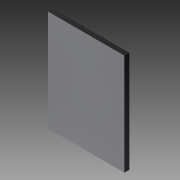
# Autodesk Inventor part: Field
Saved by Autodesk Inventor 2015 (Build 190159000, 159)
## iProperties
Created: 2016-02-20
Part Number: Field
Material: Generic
Document SubType Name: Modeling
Designer: 23902
Density: 1 g/cm^3
Appearance: Default
Author: 23902
Autodesk Inventor part; units mm, degrees
ref_plane "YZ Plane" through (0, 0, 0) normal (1, 0, 0) x (0, 1, 0)
ref_plane "XZ Plane" through (0, 0, 0) normal (0, 1, 0) x (-1, 0, 0)
ref_plane "XY Plane" through (0, 0, 0) normal (0, 0, 1) x (1, 0, 0)
sketch "Sketch1" plane through (0, 0, 0) normal (0, 1, 0) x (-1, 0, 0)
  line L0 (-910, 1215) -> (910, 1215)
  line L1 (910, 1215) -> (910, -1215)
  line L2 (910, -1215) -> (-910, -1215)
  line L3 (-910, -1215) -> (-910, 1215)
  line L4 (-910, 1215) -> (910, -1215) construction
  line L5 (910, 1215) -> (-910, -1215) construction
  point P0 (0, 0)
  dimension "d0" = 1820
  dimension "d1" = 2430
  constraints: 12 end point, 2 midpoint, 2 parallel, 1 horizontal, 1 perpendicular
  measures "d0" distance of L0.start L0.end
  measures "d1" distance of L0.end L1.end
extrude "Extrusion1" add sketch "Sketch1" along normal blind 20
sketch "Sketch2" plane through (0, 20, 0) normal (0, 1, 0) x (1, 0, 0)
  point P0 (0, 0)
sketch "Sketch3" plane through (0, 0, 0) normal (0, -1, 0) x (1, 0, 0)
  line L0 (910, 1215) -> (-910, 1215) projected
  line L1 (-910, 1215) -> (-910, -1215) projected
  line L2 (-910, -1215) -> (910, -1215) projected
  line L3 (910, -1215) -> (910, 1215) projected
  line L4 (910, 1215) -> (910, 1235)
  line L5 (910, 1235) -> (930, 1235)
  line L6 (-910, -1215) -> (-930, -1215)
  line L7 (-930, -1215) -> (-930, -1235)
  line L8 (-930, -1235) -> (930, -1235)
  line L9 (930, -1235) -> (930, 1235)
  line L10 (930, 1235) -> (-930, 1235)
  line L11 (-930, 1235) -> (-930, -1235)
  point P0 (0, 0)
  dimension "d4" = 20
  dimension "d5" = 20
  dimension "d6" = 20
  dimension "d7" = 20
  constraints: 16 end point, 3 perpendicular, 2 horizontal, 2 parallel, 1 vertical
  measures "d4" distance of L0.start L4.end
  measures "d5" distance of L4.end L5.end
  measures "d6" distance of L1.end L6.end
  measures "d7" distance of L6.end L7.end
extrude "Extrusion2" add sketch "Sketch3" against normal blind 120 contours L4 L5 L9 L8 L7 L6 L2 L3 | L0 L1 L6 L11 L10 L4
sketch "Sketch6" plane through (0, 20, 0) normal (0, 1, 0) x (1, 0, 0)
  line L0 (910, -1215) -> (-910, -1215) projected
  line L1 (225, -915) -> (245, -915)
  line L2 (245, -915) -> (245, -1215)
  line L3 (225, -915) -> (225, -989)
  line L4 (225, -989) -> (-225, -989)
  line L5 (-225, -1215) -> (-245, -1215)
  line L6 (-245, -1215) -> (-245, -915)
  line L7 (-245, -915) -> (-225, -915)
  line L8 (-225, -915) -> (-225, -989)
  line L9 (-225, -1009) -> (225, -1009)
  line L10 (225, -1009) -> (225, -1215)
  line L11 (-225, -1009) -> (-225, -1215)
  line L12 (245, -1215) -> (225, -1215)
  line L13 (225, 915) -> (245, 915)
  line L14 (245, 915) -> (245, 1215)
  line L15 (225, 915) -> (225, 989)
  line L16 (225, 989) -> (-225, 989)
  line L17 (-225, 1215) -> (-245, 1215)
  line L18 (-245, 1215) -> (-245, 915)
  line L19 (-245, 915) -> (-225, 915)
  line L20 (-225, 915) -> (-225, 989)
  line L21 (-225, 1009) -> (225, 1009)
  line L22 (225, 1009) -> (225, 1215)
  line L23 (-225, 1009) -> (-225, 1215)
  line L24 (245, 1215) -> (225, 1215)
  point P0 (0, 0)
  dimension "d22" = 20
  dimension "d23" = 74
  dimension "d24" = 450
  dimension "d25" = 20
  dimension "d26" = 20
  constraints: 48 end point, 5 perpendicular, 4 point on line, 3 vertical, 1 collinear, 1 parallel
  measures "d22" distance of L1.start L1.end
  measures "d23" distance of L1.start L3.end
  measures "d24" distance of L3.end L4.end
  measures "d25" distance of L5.start L5.end
  measures "d26" distance of L4.end L9.start
extrude "Extrusion3" add sketch "Sketch6" along normal blind 140 contours L0 L10 L9 L11 L6 L7 L8 L4 L3 L1 L2 | L15 L16 L20 L19 L18 L17 L23 L21 L22 L24 L14 L13
sketch "Sketch7" plane through (0, 160, 0) normal (0, 1, 0) x (1, 0, 0)
  line L0 (225, -915) -> (225, -989) projected
  line L1 (225, -989) -> (-225, -989) projected
  line L2 (-225, -989) -> (-225, -915) projected
  line L3 (-225, -915) -> (-245, -915) projected
  line L4 (-245, -915) -> (-245, -1215) projected
  line L5 (-245, -1215) -> (-225, -1215) projected
  line L6 (-225, -1215) -> (-225, -1009) projected
  line L7 (-225, -1009) -> (225, -1009) projected
  line L8 (225, -1009) -> (225, -1215) projected
  line L9 (225, -1215) -> (245, -1215) projected
  line L10 (245, -1215) -> (245, -915) projected
  line L11 (245, -915) -> (225, -915) projected
  line L12 (-225, 989) -> (225, 989) projected
  line L13 (225, 989) -> (225, 915) projected
  line L14 (225, 915) -> (245, 915) projected
  line L15 (245, 915) -> (245, 1215) projected
  line L16 (245, 1215) -> (225, 1215) projected
  line L17 (225, 1215) -> (225, 1009) projected
  line L18 (225, 1009) -> (-225, 1009) projected
  line L19 (-225, 1009) -> (-225, 1215) projected
  line L20 (-225, 1215) -> (-245, 1215) projected
  line L21 (-245, 1215) -> (-245, 915) projected
  line L22 (-245, 915) -> (-225, 915) projected
  line L23 (-225, 915) -> (-225, 989) projected
  line L24 (245, -1215) -> (245, -915) projected
  line L25 (-245, -915) -> (245, -915)
  line L26 (245, -915) -> (245, -1009)
  line L27 (245, -1009) -> (-245, -1009)
  line L28 (-245, -1009) -> (-245, -915)
  line L29 (245, 915) -> (245, 1215) projected
  line L30 (245, 1009) -> (-245, 1009)
  line L31 (-245, 1009) -> (-245, 915)
  line L32 (-245, 915) -> (245, 915)
  line L33 (245, 915) -> (245, 1009)
  point P0 (0, 0)
  constraints: 16 end point, 4 parallel, 2 horizontal, 2 perpendicular, 2 point on line
extrude "Extrusion4" add sketch "Sketch7" along normal blind 20 contours L11 L10 L27 L7 L4 L3 L2 L1 L0 | L0 L1 L2 L25 | L23 L22 L21 L30 L18 L15 L14 L13 L12 | L12 L13 L32 L23
body "Solid1"
